Autodesk Fusion 360 part; units mm, degrees
(part 2 of 2)
  arc A50 (5.693, 9.2091) -> (5.1337, 9.8756) centre (0, 5) ccw
  spline S23 degree 3 poles (4.7267, 7.4641) (4.8903, 7.5556) (4.9658, 7.6635) (5.0566, 7.7769) (5.3522, 8.1464) (5.5551, 8.6214) (5.677, 9.141) (5.6824, 9.1637) (5.6877, 9.1864) (5.693, 9.2091) knots 0 0 0 0 0.234809 0.234809 0.234809 1 1 1 1.034527 1.034527 1.034527 1.034527
  line L29 (4.2264, 7.1841) -> (4.7267, 7.4641)
  arc A51 (4.2264, 7.1841) -> (3.9807, 6.5092) centre (4.495, 6.7042) ccw
  arc A52 (4.0195, 6.4027) -> (3.9807, 6.5092) centre (0, 5) ccw
  arc A53 (4.0195, 6.4027) -> (4.6415, 6.0436) centre (4.5388, 6.5839) ccw
  line L30 (5.2047, 6.1507) -> (4.6415, 6.0436)
  spline S24 degree 3 poles (5.2047, 6.1507) (5.3889, 6.1857) (5.5161, 6.1516) (5.6585, 6.1231) (6.1225, 6.03) (6.5833, 5.7966) (7.0107, 5.4769) (7.0293, 5.463) (7.048, 5.449) (7.0666, 5.4351) knots 0 0 0 0 0.234809 0.234809 0.234809 1 1 1 1.034527 1.034527 1.034527 1.034527
  arc A54 (7.0666, 4.5649) -> (7.0666, 5.4351) centre (0, 5) ccw
  spline S25 degree 3 poles (5.2047, 3.8493) (5.3889, 3.8143) (5.5161, 3.8484) (5.6585, 3.8769) (6.1225, 3.97) (6.5833, 4.2034) (7.0107, 4.5231) (7.0293, 4.537) (7.048, 4.551) (7.0666, 4.5649) knots 0 0 0 0 0.234809 0.234809 0.234809 1 1 1 1.034527 1.034527 1.034527 1.034527
  line L31 (4.6415, 3.9564) -> (5.2047, 3.8493)
  arc A55 (4.6415, 3.9564) -> (4.0195, 3.5973) centre (4.5388, 3.4161) ccw
  arc A56 (3.9807, 3.4908) -> (4.0195, 3.5973) centre (0, 5) ccw
  arc A57 (3.9807, 3.4908) -> (4.2264, 2.8159) centre (4.495, 3.2958) ccw
  line L32 (4.7267, 2.5359) -> (4.2264, 2.8159)
  spline S26 degree 3 poles (4.7267, 2.5359) (4.8903, 2.4444) (4.9658, 2.3365) (5.0566, 2.2231) (5.3522, 1.8536) (5.5551, 1.3786) (5.677, 0.859) (5.6824, 0.8363) (5.6877, 0.8136) (5.693, 0.7909) knots 0 0 0 0 0.234809 0.234809 0.234809 1 1 1 1.034527 1.034527 1.034527 1.034527
  arc A58 (5.1337, 0.1244) -> (5.693, 0.7909) centre (0, 5) ccw
  spline S27 degree 3 poles (3.2474, 0.773) (3.366, 0.6278) (3.4853, 0.5721) (3.6128, 0.5025) (4.028, 0.2755) (4.531, 0.1581) (5.0639, 0.1283) (5.0872, 0.127) (5.1104, 0.1257) (5.1337, 0.1244) knots 0 0 0 0 0.234809 0.234809 0.234809 1 1 1 1.034527 1.034527 1.034527 1.034527
  line L33 (2.8848, 1.2171) -> (3.2474, 0.773)
  arc A59 (2.8848, 1.2171) -> (2.1775, 1.3418) centre (2.4588, 0.8692) ccw
  arc A60 (2.0793, 1.2851) -> (2.1775, 1.3418) centre (0, 5) ccw
  arc A61 (2.0793, 1.2851) -> (1.8337, 0.6102) centre (2.348, 0.8052) ccw
  line L34 (2.037, 0.0742) -> (1.8337, 0.6102)
  spline S28 degree 3 poles (2.037, 0.0742) (2.1035, -0.1012) (2.092, -0.2323) (2.0886, -0.3775) (2.0775, -0.8506) (1.9277, -1.3449) (1.6871, -1.8213) (1.6766, -1.8421) (1.6661, -1.8629) (1.6556, -1.8837) knots 0 0 0 0 0.234809 0.234809 0.234809 1 1 1 1.034527 1.034527 1.034527 1.034527
  arc A62 (0.7986, -2.0348) -> (1.6556, -1.8837) centre (0, 5) ccw
  spline S29 degree 3 poles (-0.2294, -0.3255) (-0.2319, -0.513) (-0.1763, -0.6323) (-0.1234, -0.7675) (0.0488, -1.2084) (0.3586, -1.6216) (0.7477, -1.987) (0.7647, -2.0029) (0.7817, -2.0189) (0.7986, -2.0348) knots 0 0 0 0 0.234809 0.234809 0.234809 1 1 1 1.034527 1.034527 1.034527 1.034527
  line L35 (-0.2217, 0.2478) -> (-0.2294, -0.3255)
  arc A63 (-0.2217, 0.2478) -> (-0.6834, 0.798) centre (-0.7717, 0.2551) ccw
  arc A64 (-0.795, 0.8177) -> (-0.6834, 0.798) centre (0, 5) ccw
  arc A65 (-0.795, 0.8177) -> (-1.417, 0.4585) centre (-0.8977, 0.2774) ccw
  line L36 (-1.6059, -0.0827) -> (-1.417, 0.4585)
  spline S30 degree 3 poles (-1.6059, -0.0827) (-1.6676, -0.2598) (-1.7607, -0.3529) (-1.8566, -0.4619) (-2.1692, -0.8173) (-2.6017, -1.0996) (-3.0923, -1.3099) (-3.1137, -1.3191) (-3.1351, -1.3282) (-3.1565, -1.3374) knots 0 0 0 0 0.234809 0.234809 0.234809 1 1 1 1.034527 1.034527 1.034527 1.034527
  arc A66 (-3.9101, -0.9023) -> (-3.1565, -1.3374) centre (0, 5) ccw
  spline S31 degree 3 poles (-3.5989, 1.0679) (-3.7213, 0.9259) (-3.7554, 0.7987) (-3.8019, 0.6611) (-3.9533, 0.2128) (-3.9815, -0.303) (-3.9184, -0.8329) (-3.9156, -0.8561) (-3.9129, -0.8792) (-3.9101, -0.9023) knots 0 0 0 0 0.234809 0.234809 0.234809 1 1 1 1.034527 1.034527 1.034527 1.034527
  line L37 (-3.2245, 1.5021) -> (-3.5989, 1.0679)
  arc A67 (-3.2245, 1.5021) -> (-3.2245, 2.2204) centre (-3.6411, 1.8612) ccw
  arc A68 (-3.2973, 2.3072) -> (-3.2245, 2.2204) centre (0, 5) ccw
  arc A69 (-3.2973, 2.3072) -> (-4.0047, 2.4319) centre (-3.7233, 1.9593) ccw
  line L38 (-4.4973, 2.1386) -> (-4.0047, 2.4319)
  spline S32 degree 3 poles (-4.4973, 2.1386) (-4.6584, 2.0427) (-4.7896, 2.0312) (-4.9331, 2.0093) (-5.401, 1.9381) (-5.9138, 1.9998) (-6.4247, 2.154) (-6.447, 2.1608) (-6.4693, 2.1675) (-6.4916, 2.1742) knots 0 0 0 0 0.234809 0.234809 0.234809 1 1 1 1.034527 1.034527 1.034527 1.034527
  arc A70 (-6.7893, 2.9919) -> (-6.4916, 2.1742) centre (0, 5) ccw
  spline S33 degree 3 poles (-5.2844, 4.3012) (-5.4695, 4.2711) (-5.5773, 4.1956) (-5.7014, 4.12) (-6.1056, 3.8739) (-6.4587, 3.497) (-6.751, 3.0504) (-6.7637, 3.0309) (-6.7765, 3.0114) (-6.7893, 2.9919) knots 0 0 0 0 0.234809 0.234809 0.234809 1 1 1 1.034527 1.034527 1.034527 1.034527
  line L39 (-4.7185, 4.3931) -> (-5.2844, 4.3012)
  arc A71 (-4.7185, 4.3931) -> (-4.2568, 4.9433) centre (-4.8068, 4.936) ccw
  arc A72 (-4.2568, 5.0567) -> (-4.2568, 4.9433) centre (0, 5) ccw
  arc A73 (-4.2568, 5.0567) -> (-4.7185, 5.6069) centre (-4.8068, 5.064) ccw
  line L40 (-5.2844, 5.6988) -> (-4.7185, 5.6069)
  spline S34 degree 3 poles (-5.2844, 5.6988) (-5.4695, 5.7289) (-5.5773, 5.8044) (-5.7014, 5.88) (-6.1056, 6.1261) (-6.4587, 6.503) (-6.751, 6.9496) (-6.7637, 6.9691) (-6.7765, 6.9886) (-6.7893, 7.0081) knots 0 0 0 0 0.234809 0.234809 0.234809 1 1 1 1.034527 1.034527 1.034527 1.034527
  arc A74 (-6.4916, 7.8258) -> (-6.7893, 7.0081) centre (0, 5) ccw
  spline S35 degree 3 poles (-4.4973, 7.8614) (-4.6584, 7.9573) (-4.7896, 7.9688) (-4.9331, 7.9907) (-5.401, 8.0619) (-5.9138, 8.0002) (-6.4247, 7.846) (-6.447, 7.8392) (-6.4693, 7.8325) (-6.4916, 7.8258) knots 0 0 0 0 0.234809 0.234809 0.234809 1 1 1 1.034527 1.034527 1.034527 1.034527
  line L41 (-4.0047, 7.5681) -> (-4.4973, 7.8614)
  arc A75 (-4.0047, 7.5681) -> (-3.2973, 7.6928) centre (-3.7233, 8.0407) ccw
  arc A76 (-3.2245, 7.7796) -> (-3.2973, 7.6928) centre (0, 5) ccw
  arc A77 (-3.2245, 7.7796) -> (-3.2245, 8.4979) centre (-3.6411, 8.1388) ccw
  line L42 (-3.5989, 8.9321) -> (-3.2245, 8.4979)
  point P0 (0, 5)
  dimension "d80" = 17.5
  dimension "d81" = 14
  dimension "d87" = 2.8
  dimension "d94" = 9.8
  dimension "d100" = 5
  dimension "d101" = 3.5
  dimension "d108" = 0.15
  constraint concentric A1 A38
  constraint concentric A38 A39
  constraint coincident P0 A1.centre
  constraint concentric A38 A40
  constraint concentric A40 A41
  measures "d80" diameter of A38
  measures "d81" diameter of A39
  measures "d87" distance of P0 L23
  measures "d94" diameter of A40
  measures "d100" diameter of A1
  measures "d101" diameter of A41
extrude "Extrude11" add sketch "Sketch5" along normal blind 5 separate body contours A0 A38 A39 S24 A54 S25 S26 A58 S27 S28 A62 S29 S30 A66 S31 S32 A70 S33 S34 A74 | A0 A38 A39 S18 A42 S19 S20 A46 S21 S22 A50 S23 A74 S35 | A0 A39 A40 S23 L29 L30 S24 | A0 A39 S23 | A0 A39 S21 L27 S22 | A0 A39 S18 S35 | A39 A40 S33 L39 L40 S34 | A40 L29 A51 A52 A53 L30 | A39 A40 S25 L31 L32 S26 | A0 A40 L27 L28 S22 | A0 A40 S18 S35 L41 L42 | A0 A39 S19 L25 L26 S20 | A39 A40 S31 L37 L38 S32 | A40 L39 A71 A72 A73 L40 | A39 A40 S27 L33 L34 S28 | A40 L31 A55 A56 A57 L32 | A40 L27 A47 A48 A49 L28 | A40 L41 A75 A76 A77 L42 | A0 A40 L25 L26 | A39 A40 S29 L35 L36 S30 | A40 L37 A67 A68 A69 L38 | A40 L33 A59 A60 A61 L34 | A40 L25 A43 A44 A45 L26 | A40 L35 A63 A64 A65 L36 makes body 2
extrude "Extrude12" add sketch "Sketch5" against normal blind 20 contours A0 A38 A39 S24 A54 S25 S26 A58 S27 S28 A62 S29 S30 A66 S31 S32 A70 S33 S34 A74 | A0 A38 A39 S18 A42 S19 S20 A46 S21 S22 A50 S23 A74 S35 | A0 A39 A40 S23 L29 L30 S24 | A0 A39 S23 | A0 A39 A74 S35 | A0 A39 S34 A74 | A0 L16 S16 A40 S23 L29 | A0 S16 A35 S17 A39 S22 S23 | A39 S24 A54 S25 | L14 S14 A31 S15 L15 A39 A40 L30 S24 S25 L31 | A39 S22 A50 S23 | A0 S4 A11 A39 S35 | A0 A11 S5 L5 A39 A40 L40 S34 | A0 L16 S16 S17 L17 A40 | A0 S16 A35 S17 | A0 A39 S21 L27 S22 | A0 L4 S4 A11 S5 L5 A40 | A0 A39 S18 S35 | A39 A40 S33 L39 L40 S34 | A0 S17 L17 A40 L28 S22 | A39 A40 S25 L31 L32 S26 | A0 L0 S0 A3 S1 L1 A39 L26 S20 S21 L27 | A39 S20 A46 S21 | A0 A40 L27 L28 S22 | A0 L4 S4 A40 S35 L41 | A39 S18 A42 S19 | A0 L2 S2 A7 S3 A39 S18 S19 L25 | A0 A40 S18 S35 L41 L42 | L6 S6 A15 S7 L7 A39 A40 L38 S32 S33 L39 | A39 S32 A70 S33 | A39 S26 A58 S27 | L12 S12 A27 S13 L13 A39 A40 L32 S26 S27 L33 | L14 S14 A31 S15 L15 A40 | A0 A39 S19 L25 L26 S20 | A0 L0 A40 L27 | A0 S3 L3 A40 S18 L42 | A39 A40 S31 L37 L38 S32 | A39 A40 S27 L33 L34 S28 | A0 L0 L1 A40 | A0 L0 S0 A3 S1 L1 | A0 L2 S2 A7 S3 | A0 L2 S3 L3 A40 | L8 S8 A19 S9 L9 A39 A40 L36 S30 S31 L37 | A39 S30 A66 S31 | A39 S28 A62 S29 | L10 S10 A23 S11 L11 A39 A40 L34 S28 S29 L35 | A0 A40 L25 L26 | A0 L1 A40 L26 | A0 L2 A40 L25 | A39 A40 S29 L35 L36 S30 | L6 S6 A15 S7 L7 A40 | L12 S12 A27 S13 L13 A40 | L8 S8 A19 S9 L9 A40 | L10 S10 A23 S11 L11 A40 bodies 2
extrude "Extrude13" add sketch "Sketch5" against normal blind 5 contours A0 A39 A40 S23 L29 L30 S24 | A0 A39 S23 | A0 L16 S16 A40 S23 L29 | A0 S16 A35 S17 A39 S22 S23 | L14 S14 A31 S15 L15 A39 A40 L30 S24 S25 L31 | A0 S4 A11 A39 S35 | A0 A11 S5 L5 A39 A40 L40 S34 | A0 L16 S16 S17 L17 A40 | A0 S16 A35 S17 | A0 A39 S21 L27 S22 | A0 L4 S4 A11 S5 L5 A40 | A0 A39 S18 S35 | A39 A40 S33 L39 L40 S34 | A0 S17 L17 A40 L28 S22 | L15 A32 A33 A34 L16 A40 L29 A51 A52 A53 L30 | A40 L29 A51 A52 A53 L30 | A39 A40 S25 L31 L32 S26 | A0 L0 S0 A3 S1 L1 A39 L26 S20 S21 L27 | A0 A40 L27 L28 S22 | A0 L4 S4 A40 S35 L41 | A0 L2 S2 A7 S3 A39 S18 S19 L25 | A0 A40 S18 S35 L41 L42 | L6 S6 A15 S7 L7 A39 A40 L38 S32 S33 L39 | A2 L0 L1 A4 A5 A6 L2 L3 A8 A9 A10 L4 L5 A12 A13 A14 L6 L7 A16 A17 A18 L8 L9 A20 A21 A22 L10 L11 A24 A25 A26 L12 L13 A28 A29 A30 L14 L15 A32 A33 A34 L16 L17 A36 A37 A40 | L12 S12 A27 S13 L13 A39 A40 L32 S26 S27 L33 | L14 S14 A31 S15 L15 A40 | A0 A39 S19 L25 L26 S20 | A0 L0 A40 L27 | A0 S3 L3 A40 S18 L42 | A39 A40 S31 L37 L38 S32 | A40 L39 A71 A72 A73 L40 | L5 A12 A13 A14 L6 A40 L39 A71 A72 A73 L40 | A2 L0 L17 A36 A37 A40 L27 A47 A48 A49 L28 | A39 A40 S27 L33 L34 S28 | L13 A28 A29 A30 L14 A40 L31 A55 A56 A57 L32 | A40 L31 A55 A56 A57 L32 | A0 L0 L1 A40 | A0 L0 S0 A3 S1 L1 | A40 L27 A47 A48 A49 L28 | L3 A8 A9 A10 L4 A40 L41 A75 A76 A77 L42 | A0 L2 S2 A7 S3 | A0 L2 S3 L3 A40 | A40 L41 A75 A76 A77 L42 | L8 S8 A19 S9 L9 A39 A40 L36 S30 S31 L37 | L10 S10 A23 S11 L11 A39 A40 L34 S28 S29 L35 | A0 A40 L25 L26 | A0 L1 A40 L26 | A0 L2 A40 L25 | A39 A40 S29 L35 L36 S30 | A40 L37 A67 A68 A69 L38 | L7 A16 A17 A18 L8 A40 L37 A67 A68 A69 L38 | L6 S6 A15 S7 L7 A40 | L11 A24 A25 A26 L12 A40 L33 A59 A60 A61 L34 | A40 L33 A59 A60 A61 L34 | L12 S12 A27 S13 L13 A40 | A40 L25 A43 A44 A45 L26 | L1 A4 A5 A6 L2 A40 L25 A43 A44 A45 L26 | A40 L35 A63 A64 A65 L36 | L9 A20 A21 A22 L10 A40 L35 A63 A64 A65 L36 | L8 S8 A19 S9 L9 A40 | L10 S10 A23 S11 L11 A40 bodies 2
extrude "Extrude14" add sketch "Sketch5" against normal blind 2.5 from surface at -2.5 contours A1 | L18 L19 L20 L21 L22 L23 | A41 bodies 2
extrude "Extrude15" cut sketch "Sketch5" against normal blind 9 contours A41 bodies 2
fillet "Fillet1'" radius 1 1 edges at (-4.5684, 19, 3.2281) on bodies 2
component "Spur Gear (9 teeth) (1)" placed x (1, 0, 0) y (0, 1, 0) z (0, 0, 1) at (0, 0, 0)
